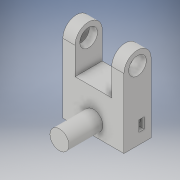
# Autodesk Inventor part: EndEffectorV2
Saved by Autodesk Inventor 2017 (Build 210142000, 142)
## iProperties
Created: 2018-10-15
Part Number: EndEffectorV2
Material: Generic
Document SubType Name: Modeling
Designer: Tom
Density: 1 g/cm^3
Appearance: Default
Author: Tom
Autodesk Inventor part; units mm, degrees
ref_plane "YZ Plane" through (0, 0, 0) normal (1, 0, 0) x (0, 1, 0)
ref_plane "XZ Plane" through (0, 0, 0) normal (0, 1, 0) x (-1, 0, 0)
sketch "Sketch15" plane through (0, 0, 0) normal (0, 1, 0) x (-1, 0, 0)
  line L0 (0, 0) -> (45, 0)
  line L1 (45, 0) -> (45, -20)
  line L2 (45, -20) -> (0, -20)
  line L3 (0, -20) -> (0, 0)
  dimension "d88" = 45
  dimension "d89" = 20
  constraints: 8 end point, 2 parallel, 1 horizontal, 1 perpendicular
  measures "d88" distance of L1.end L2.end
  measures "d89" distance of L0.end L1.end
extrude "Extrusion11" add sketch "Sketch15" along normal blind 20
sketch "Sketch16" plane through (-45, 0, 0) normal (0, 0, 1) x (1, 0, 0)
  line L0 (45, 0) -> (45, 20) projected
  line L1 (0, 20) -> (45, 20) projected
  circle A0 centre (22.5, 10) radius 7
  dimension "d92" = 14
  dimension "d93" = 10
  dimension "d94" = 22.5
  constraints: 1 centre point
  measures "d92" diameter of A0
  measures "d93" distance from line of L1 A0.centre
  measures "d94" distance from line of L0 A0.centre
extrude "Extrusion12" add sketch "Sketch16" along normal blind 25
sketch "Sketch17" plane through (0, 0, 0) normal (1, 0, 0) x (0, 0, -1)
  line L0 (20, 0) -> (20, 20) projected
  line L1 (0, 0) -> (0, 20) projected
  line L2 (-25, 17) -> (-25, 3) projected
  line L3 (0, 3) -> (0, 17) projected
  line L4 (-25, 10) -> (20, 10) construction
  line L5 (0, 20) -> (20, 20)
  line L6 (20, 20) -> (20, 51)
  line L7 (0, 51) -> (0, 20)
  arc A0 (20, 51) -> (0, 51) centre (10, 51) ccw
  circle A1 centre (10, 51) radius 6.5 construction
  dimension "d98" = 41
  dimension "d99" = 13
  constraints: 8 end point, 2 centre point, 2 collinear, 2 midpoint, 2 point on circle, 1 coincident, 1 horizontal, 1 parallel, 1 perpendicular
  measures "d98" distance from line of L4 A0.centre
  measures "d99" diameter of A1
extrude "Extrusion13" add sketch "Sketch17" against normal up to surface (45 mm away)
sketch "Sketch18" plane through (0, 0, -20) normal (0, 0, -1) x (-1, 0, 0)
  line L0 (0, 61) -> (45, 61) projected
  line L1 (9, 31) -> (36, 31)
  line L2 (36, 31) -> (36, 61)
  line L3 (36, 61) -> (9, 61)
  line L4 (9, 61) -> (9, 31)
  line L5 (45, 61) -> (45, 51) projected
  line L6 (0, 61) -> (0, 51) projected
  line L7 (0, 51) -> (45, 51) projected
  line L8 (14.6068, 31.9261) -> (20.6068, 31.9261)
  line L9 (20.6068, 31.9261) -> (20.6068, 53.9261)
  line L10 (20.6068, 53.9261) -> (14.6068, 53.9261)
  line L11 (14.6068, 53.9261) -> (14.6068, 31.9261)
  line L12 (20.6068, 25.659) -> (25.6068, 25.659)
  line L13 (25.6068, 25.659) -> (25.6068, 59.659)
  line L14 (25.6068, 59.659) -> (20.6068, 59.659)
  line L15 (20.6068, 59.659) -> (20.6068, 25.659)
  point P0 (40, 20)
  point P1 (0, 20)
  dimension "d105" = 30
  dimension "d106" = 9
  dimension "d107" = 9
  dimension "d116" = 20
  dimension "d117" = 6
  dimension "d118" = 22
  dimension "d119" = 5
  dimension "d120" = 34
  dimension "d121" = 10.3932
  dimension "d122" = 11.6068
  constraints: 24 end point, 6 parallel, 3 horizontal, 3 perpendicular, 1 point on line
  measures "d105" distance between parallel lines of L1 L0
  measures "d106" distance between parallel lines of L2 L5
  measures "d107" distance between parallel lines of L6 L4
  measures "d116" distance between parallel lines of L1 L7
  measures "d117" distance of L10.end L9.end
  measures "d118" distance of L9.end L8.end
  measures "d119" distance of L14.end L13.end
  measures "d120" distance of L13.end L12.end
  measures "d121" distance between parallel lines of L2 L13
  measures "d122" distance between parallel lines of L4 L15
extrude "Extrusion14" cut sketch "Sketch18" against normal through all contours L0 L2 L7 L13 L14 L15 L10 L11 L4 | L7 L11 L8 L15 L1 L4 | L2 L1 L13 L7 | L11 L10 L9 L7 | L7 L9 L8 L11 | L13 L1 L15 L9 L7 | L7 L9 L15 L14 L13
sketch "Sketch19" plane through (-36, 31, -20) normal (1, 0, 0) x (0, 0, -1)
  arc A0 (0, 20) -> (-20, 20) centre (-10, 20) ccw projected
  circle A1 centre (-10, 20) radius 6.5
  point P0 (-20, -31)
  point P1 (0, 22.9052)
  dimension "d110" = 13
  constraints: 1 centre point, 1 coincident, 1 other
  measures "d110" diameter of A1
extrude "Extrusion15" cut sketch "Sketch19" against normal blind 6
sketch "Sketch20" plane through (-9, 31, -20) normal (-1, 0, 0) x (0, 0, 1)
  arc A0 (20, 20) -> (0, 20) centre (10, 20) ccw projected
  circle A1 centre (10, 20) radius 6.5
  point P0 (20, -31)
  point P1 (0, 22.9052)
  dimension "d113" = 13
  constraints: 1 centre point, 1 coincident, 1 other
  measures "d113" diameter of A1
extrude "Extrusion16" cut sketch "Sketch20" against normal through all
sketch "Sketch21" plane through (0, 0, -20) normal (0, 0, -1) x (-1, 0, 0)
  line L0 (36, 31) -> (9, 31) projected
  line L1 (45, 0) -> (30, 0)
  line L2 (30, 0) -> (30, 31)
  line L3 (30, 31) -> (45, 31)
  line L4 (45, 31) -> (45, 0)
  line L5 (0, 0) -> (15, 0)
  line L6 (15, 0) -> (15, 31)
  line L7 (15, 31) -> (0, 31)
  line L8 (0, 31) -> (0, 0)
  line L9 (45, 0) -> (0, 0) projected
  line L10 (9, 31) -> (36, 31) projected
  line L11 (22.5, 31) -> (22.5, 0) construction
  point P0 (6, 19.5)
  point P1 (39, 19.5)
  dimension "d123" = 15
  dimension "d124" = 15
  dimension "d132" = 16.5
  dimension "d133" = 16.5
  constraints: 18 end point, 4 parallel, 2 horizontal, 2 midpoint, 2 perpendicular, 2 point on line
  measures "d123" distance of L6.end L7.end
  measures "d124" distance of L2.end L3.end
  measures "d132" distance from line of L11 point (39, 19.5)
  measures "d133" distance from line of point (6, 19.5) L11
extrude "Extrusion17" [suppressed]
sketch "Sketch22" plane through (-45, 0, 0) normal (-1, 0, 0) x (0, 0, 1)
  line L0 (0, 0) -> (-20, 0) projected
  line L1 (-30, 23) -> (-20, 23)
  line L2 (-20, 23) -> (-20, 0)
  line L3 (-20, 0) -> (-30, 0)
  line L4 (-30, 0) -> (-30, 23)
  point P0 (-30, 0)
  constraints: 9 end point, 2 parallel, 1 horizontal, 1 perpendicular
extrude "Extrusion18" [suppressed]
sketch "Sketch23" plane through (0, 51, -10) normal (1, 0, 0) x (0, 0, -1)
  line L0 (10, -43) -> (10, -20) projected
  line L1 (20, -43) -> (10, -43)
  line L2 (10, -43) -> (10, -20)
  line L3 (10, -20) -> (20, -20)
  line L4 (20, -20) -> (20, -43)
  constraints: 8 end point, 2 parallel, 1 horizontal, 1 perpendicular
extrude "Extrusion19" [suppressed]
sketch "Sketch24" plane through (12, 43, -10) normal (1, 0, 0) x (0, 0, -1)
  line L0 (10, -20) -> (10, -43) projected
  line L1 (20, -20) -> (10, -20)
  line L2 (10, -20) -> (10, -31.5)
  line L3 (10, -31.5) -> (20, -31.5)
  line L4 (20, -31.5) -> (20, -20)
  point P0 (-10, -43)
  constraints: 8 end point, 2 parallel, 1 horizontal, 1 midpoint, 1 perpendicular
revolve "Revolution1" [suppressed]
sketch "Sketch25" plane through (0, 0, -30) normal (0, 0, -1) x (-1, 0, 0)
  line L0 (15, 0) -> (-12, 0) projected
  line L1 (15, 0) -> (15, 23) projected
  line L2 (15, 23) -> (-12, 23) projected
  arc A0 (-12, 23) -> (-12, 0) centre (-12, 11.5) ccw projected
  point P0 (0, 0)
  point P1 (-3.6176, 11.5)
  point P2 (49.207, 11.5)
sketch "Sketch26" plane through (0, 0, -20) normal (0, 0, -1) x (-1, 0, 0)
  line L0 (0, 0) -> (0, 51) projected
  line L1 (45, 0) -> (0, 0) projected
  line L2 (45, 0) -> (45, 51) projected
  line L3 (-6.2428, 12) -> (58.3359, 12)
  point P0 (6, 12)
  point P1 (39, 12)
  dimension "d134" = 12
  dimension "d135" = 6
  dimension "d136" = 33
  dimension "d137" = 6
  constraints: 2 end point, 2 point on line, 1 horizontal
  measures "d134" distance between parallel lines of L1 L3
  measures "d135" distance from line of L2 point (39, 12)
  measures "d136" distance of point (6, 12) point (39, 12)
  measures "d137" distance from line of L0 point (6, 12)
hole "Hole2" at (-39, 12, -20) direction (0, 0, 1) diameter 4 depth 6 tip angle 118
sketch "Sketch27" plane through (0, 0, 0) normal (1, 0, 0) x (0, 0, -1)
  line L0 (0, 10) -> (0, 14) projected
  line L1 (20, 14) -> (20, 10) projected
  line L2 (15, 16) -> (11, 16)
  line L3 (11, 16) -> (11, 8)
  line L4 (11, 8) -> (15, 8)
  line L5 (15, 8) -> (15, 16)
  line L6 (15, 12) -> (11, 12)
  line L7 (20, 14) -> (20, 10) projected
  line L8 (0, 0) -> (0, 51) projected
  line L9 (20, 14) -> (20, 10) projected
  line L10 (20, 31) -> (20, 51) projected
  line L11 (20, 0) -> (20, 51) projected
  line L12 (20, 0) -> (20, 51) projected
  line L13 (20, 51) -> (20, 31) projected
  line L14 (20, 14) -> (20, 10) projected
  line L15 (20, 12) -> (0, 12)
  dimension "d145" = 8
  dimension "d147" = 4
  dimension "d160" = 5
  constraints: 12 end point, 3 midpoint, 2 parallel, 2 perpendicular, 1 collinear, 1 horizontal, 1 point on line
  measures "d145" distance between parallel lines of L4 L2
  measures "d147" distance between parallel lines of L5 L3
  measures "d160" distance between parallel lines of L11 L5
extrude "Extrusion20" cut sketch "Sketch27" against normal blind 12
sketch "Sketch28" plane through (0, 0, -20) normal (0, 0, -1) x (-1, 0, 0)
  line L0 (0, 0) -> (0, 51) projected
  line L1 (5, 12) -> (7.5, 12) construction
  line L2 (5, 10) -> (7.5, 10)
  line L3 (7.5, 14) -> (5, 14)
  arc A0 (5, 14) -> (5, 10) centre (5, 12) ccw
  arc A1 (7.5, 10) -> (7.5, 14) centre (7.5, 12) ccw
  point P0 (6.25, 12)
  dimension "d150" = 5
  dimension "d151" = 2.5
  constraints: 8 end point, 4 point on circle, 4 tangent, 2 centre point, 1 horizontal, 1 midpoint, 1 parallel
  measures "d150" distance from line of L0 L1.start
  measures "d151" distance of L1.start L1.end
extrude "Extrusion21" cut sketch "Sketch28" against normal up to surface (9 mm away)
sketch "Sketch29" plane through (-45, 0, -20) normal (-1, 0, 0) x (0, 0, 1)
  line L0 (0, 0) -> (0, 51) projected
  line L1 (20, 0) -> (20, 43)
  line L2 (0, 10) -> (0, 14)
  line L3 (20, 14) -> (20, 10)
  line L4 (9, 16) -> (5, 16)
  line L5 (5, 16) -> (5, 8)
  line L6 (5, 8) -> (9, 8)
  line L7 (9, 8) -> (9, 16)
  line L8 (9, 12) -> (5, 12)
  line L9 (20, 14) -> (20, 10)
  line L10 (20, 12) -> (0, 12) construction
  line L11 (0, 10) -> (0, 14) projected
  dimension "d154" = 8
  dimension "d156" = 4
  dimension "d157" = 5
  constraints: 20 end point, 4 midpoint, 2 parallel, 1 collinear, 1 horizontal, 1 perpendicular
  measures "d154" distance between parallel lines of L6 L4
  measures "d156" distance between parallel lines of L7 L5
  measures "d157" distance between parallel lines of L0 L5
extrude "Extrusion22" cut sketch "Sketch29" against normal blind 12
ref_plane "Work Plane2" through (-22.5, 3, 0) normal (0, 1, 0) x (-1, 0, 0)
sketch "Sketch30" plane through (-22.5, 3, 0) normal (0, 1, 0) x (-1, 0, 0)
  line L0 (7, 25) -> (-7, 25) projected
  line L1 (-7, 0) -> (7, 0) projected
  point P0 (-22.5, 0)
  point P1 (0, 17)
  dimension "d161" = 8
  measures "d161" distance from line of L0 point (0, 17)
hole "Hole3" at (-22.5, 3, 17) direction (0, 1, 0) diameter 3 depth 8 tip angle 118
equation "\"d106\" = d107"
equation "\"d124\" = d123"
body "Solid2"
